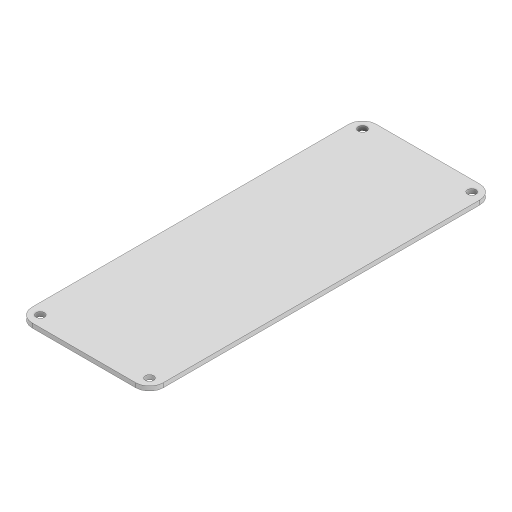
# Autodesk Inventor part: Control_PCB
Saved by Autodesk Inventor 2023 (Build 270158000, 158)
## iProperties
Created: 2026-04-14
Part Number: Control_PCB
Material: Generic
Document SubType Name: Modeling
Designer: ferrerx
Density: 1 g/cm^3
Appearance: Default
Author: ferrerx
Autodesk Inventor part; units mm, degrees
ref_plane "YZ Plane" through (0, 0, 0) normal (1, 0, 0) x (0, 1, 0)
ref_plane "XZ Plane" through (0, 0, 0) normal (0, 1, 0) x (-1, 0, 0)
ref_plane "XY Plane" through (0, 0, 0) normal (0, 0, 1) x (1, 0, 0)
sketch "Sketch1" plane through (0, 0, 0) normal (0, 1, 0) x (-1, 0, 0)
  line L0 (-24, 63) -> (24, 63)
  line L1 (24, 63) -> (24, -63)
  line L2 (24, -63) -> (-24, -63)
  line L3 (-24, -63) -> (-24, 63)
  line L4 (-24, 63) -> (24, -63) construction
  line L5 (24, 63) -> (-24, -63) construction
  line L6 (-20, 59) -> (20, 59) construction
  line L7 (20, 59) -> (20, -59) construction
  line L8 (20, -59) -> (-20, -59) construction
  line L9 (-20, -59) -> (-20, 59) construction
  line L10 (-20, 59) -> (20, -59) construction
  line L11 (20, 59) -> (-20, -59) construction
  circle A0 centre (20, 59) radius 1.55
  circle A1 centre (20, -59) radius 1.55
  circle A2 centre (-20, -59) radius 1.55
  circle A3 centre (-20, 59) radius 1.55
  point P0 (0, 0)
  dimension "d0" = 126
  dimension "d1" = 48
  dimension "d2" = 3.1
  dimension "d3" = 4
  dimension "d4" = 4
  dimension "d5" = 3.1
  dimension "d6" = 3.1
  dimension "d7" = 3.1
  constraints: 24 end point, 4 centre point, 4 coincident, 4 midpoint, 4 parallel, 2 horizontal, 2 perpendicular
  measures "d0" distance of L0.end L1.end
  measures "d1" distance of L0.start L0.end
  measures "d2" diameter of A0
  measures "d3" distance between parallel lines of L1 L7
  measures "d4" distance between parallel lines of L0 L6
  measures "d5" diameter of A3
  measures "d6" diameter of A2
  measures "d7" diameter of A1
extrude "Extrusion1" add sketch "Sketch1" along normal blind 1.6
fillet "Fillet1" radius 5 4 edges at (24, 0.8, -63) (-24, 0.8, -63) (24, 0.8, 63) (-24, 0.8, 63)
equation "\"d5\" = d2"
equation "\"d6\" = d2"
equation "\"d7\" = d2"
body "Solid1"
